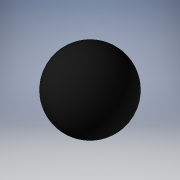
# Autodesk Inventor part: 6000DDU Ball
Saved by Autodesk Inventor 2023 (Build 270158000, 158)
## iProperties
Created: 2023-07-21
Part Number: 6000DDU Ball
Material: Generic
Catalog Web Link: www.cadenas.de
Description: contact_sealed_type_dd_ddu_B-NSK
Vendor: NSK_RB
Document SubType Name: Modeling
Designer: psAdmin
Manufacturer: NSK_RB
Mass: 0.0335103 g
Surface Area: 0.502655 cm^2
Volume: 0.0335103 cm^3
Density: 1 g/cm^3
Appearance: PSOLRGB-128-128-128
Category: PARTsolutions
Company: NSK_RB
PSOL_IDENT_0: {$CADENAS_DATA/23d-libs/nsk_rb/roller_bearings/deep_groove_bb/single_row_dgbb/contact_sealed_type_dd
PSOL_IDENT_1: _ddu_2_b.prj},186 {VTYP=3D},{NB=6000DDU Ball},{LINA=6000DDU Ball},{NN=contact_sealed_type_dd_ddu_B},
PSOL_IDENT_2: {DATE=15.09.2022 00:32:48},{GEOMDATE=18.05.2018 11:37:08},{VERSION=},{LINEID=30},{WBVAR=},{WBNUMERIC=
PSOL_IDENT_3: }  {NB=6000DDU Ball},{LINA=6000DDU Ball},{KT=DUMMY},{IDNR=},{STAN=Standard},{ORDER=6000DDU},{SD=10},
PSOL_IDENT_4: {X=10},{DI1=14.57},{DI2=13.2},{SDE1=21.50},{SDE2=23.00},{D=26},{DD=26},{B=8},{R=0.3},{CR1=4550},{COR
PSOL_IDENT_5: 1=1970},{CR2=465},{COR2=201},{FO=12.4},{LG=22000},{A=1.35},{BB=0.87},{DD1=24.50},{RO=0.20},{RN=0.3},
PSOL_IDENT_6: {DD2=28.7},{F=0.84},{DAM1=12.0},{DA1=13.0},{DA2=24.0},{RA=0.3},{DX=29.4},{CY=1.9},{MASS=0.018},{SC=1
PSOL_IDENT_7: }
NB: 6000DDU Ball
NN: contact_sealed_type_dd_ddu_B
NT: NSK
NBSYN: $ORDER. Ball
LINA: 6000DDU Ball
CATALOG: NSK Rolling Bearing
STAN: Standard
ORDER: 6000DDU
SD: 10
X: 10
DI1: 14.57
DI2: 13.2
SDE1: 21.5
SDE2: 23
D: 26
DD: 26
B: 8
R: 0.3
CR1: 4550
COR1: 1970
CR2: 465
COR2: 201
FO: 12.4
LG: 22000
A: 1.35
BB: 0.87
DD1: 24.5
RO: 0.2
RN: 0.3
DD2: 28.7
F: 0.84
DAM1: 12
DA1: 13
DA2: 24
RA: 0.3
DX: 29.4
CY: 1.9
MASS: 0.018
SC: 1
SUPPLIER: NSK_RB
ARTICLENO: 6000DDU Ball
BOMINFO: 6000DDU Ball
CREATOR: CADENAS GmbH
Title: 6000DDU Ball
Author: Cadenas PARTsolutions
Comments: NSK
Autodesk Inventor part; units mm, degrees
sketch "Sketch_1" plane through (0, 0, 0) normal (0, 0, 1) x (1, 0, 0)
  line L0 (2, 0) -> (-2, 0)
  arc A0 (2, 0) -> (-2, 0) centre (0, 0) ccw
  line L1 (2, 0) -> (-2, 0)
  constraints: 4 end point, 2 point on circle, 1 centre point
revolve "Revolution1" add sketch "Sketch_1" angle 360 about axis through (2, 0, 0) along (1, 0, 0)
ref_plane "ip_cst_2_b_1_XY" through (0, 0, 0) normal (1, 0, 0) x (0, 0, -1)
ref_plane "ip_cst_2_b_1_YZ" through (0, 0, 0) normal (0, 0, -1) x (0, 1, 0)
ref_plane "ip_cst_2_b_1_ZX" through (0, 0, 0) normal (0, 1, 0) x (1, 0, 0)
body "Solid1"
